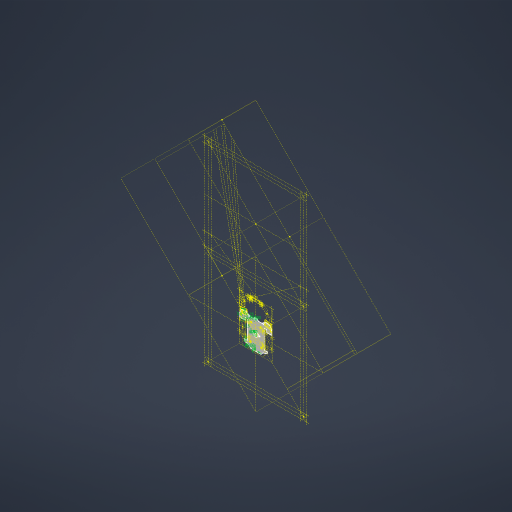
# Autodesk Inventor part: circuit
Saved by Autodesk Inventor 2023.5 (Build 275446000, 446)
## iProperties
Created: 2025-01-11
Part Number: circuit
Material: 一般
Document SubType Name: Modeling
Designer: IshiiLabHonda
Density: 1 g/cm^3
Appearance: 既定
Author: IshiiLabHonda
Autodesk Inventor part; units mm, degrees
ref_plane "YZ Plane" through (0, 0, 0) normal (1, 0, 0) x (0, 1, 0)
ref_plane "XZ Plane" through (0, 0, 0) normal (0, 1, 0) x (-1, 0, 0)
ref_plane "XY Plane" through (0, 0, 0) normal (0, 0, 1) x (1, 0, 0)
derived "chassis.ipt"
sketch "スケッチ1" plane through (0, 0, 0) normal (0, 0, 1) x (1, 0, 0)
  line L0 (0, 0) -> (0, 1) construction
  line L1 (0, 0) -> (1, 0) construction
  line L2 (-90, 90) -> (90, 90) construction
  line L3 (90, 90) -> (90, -90) construction
  line L4 (90, -90) -> (-90, -90) construction
  line L5 (-90, -90) -> (-90, 90) construction
  line L6 (-90, -90) -> (90, 90) construction
  line L7 (-90, 90) -> (90, -90) construction
  line L8 (-84, 96) -> (-84, 84) construction
  line L9 (-84, 84) -> (-96, 84) construction
  line L10 (-96, 84) -> (-96, 96) construction
  line L11 (-96, 96) -> (-84, 84) construction
  line L12 (-84, 96) -> (-96, 84) construction
  line L13 (-96, 96) -> (-84, 96) construction
  line L14 (-96, -96) -> (-96, -84) construction
  line L15 (-84, -96) -> (-96, -96) construction
  line L16 (-96, -96) -> (-84, -84) construction
  line L17 (-96, -84) -> (-84, -96) construction
  line L18 (-84, -84) -> (-84, -96) construction
  line L19 (-96, -84) -> (-84, -84) construction
  line L20 (96, -96) -> (84, -96) construction
  line L21 (96, -84) -> (96, -96) construction
  line L22 (96, -96) -> (84, -84) construction
  line L23 (84, -96) -> (96, -84) construction
  line L24 (84, -84) -> (96, -84) construction
  line L25 (84, -96) -> (84, -84) construction
  line L26 (96, 96) -> (96, 84) construction
  line L27 (84, 96) -> (96, 96) construction
  line L28 (96, 96) -> (84, 84) construction
  line L29 (96, 84) -> (84, 96) construction
  line L30 (84, 84) -> (84, 96) construction
  line L31 (96, 84) -> (84, 84) construction
  line L32 (-84, 84) -> (-84, -84) construction
  line L33 (-96, 84) -> (-96, -84) construction
  line L34 (-84, -84) -> (84, -84) construction
  line L35 (-84, -96) -> (84, -96) construction
  line L36 (96, 84) -> (96, -84) construction
  line L37 (84, 84) -> (84, -84) construction
  line L38 (-84, 96) -> (84, 96) construction
  line L39 (-84, 84) -> (84, 84) construction
  line L40 (-19, 15) -> (19, 15) construction
  line L41 (19, 15) -> (19, -15) construction
  line L42 (19, -15) -> (-19, -15) construction
  line L43 (-19, -15) -> (-19, 15) construction
  line L44 (-19, 15) -> (19, -15) construction
  line L45 (19, 15) -> (-19, -15) construction
  line L46 (-30.25, 11.5) -> (-19, 11.5) construction
  line L47 (-19, -11.5) -> (-30.25, -11.5) construction
  line L48 (-30.25, -11.5) -> (-30.25, 11.5) construction
  line L49 (-30.25, 11.5) -> (-19, -11.5) construction
  line L50 (-19, 11.5) -> (-30.25, -11.5) construction
  line L51 (19, 11.5) -> (30.25, -11.5) construction
  line L52 (19, -11.5) -> (30.25, -11.5) construction
  line L53 (30.25, -11.5) -> (30.25, 11.5) construction
  line L54 (30.25, 11.5) -> (19, 11.5) construction
  line L55 (30.25, 11.5) -> (19, -11.5) construction
  line L56 (-19, -10) -> (19, -10) construction
  line L57 (-19, -12.5) -> (19, -12.5) construction
  line L58 (-19, 12.5) -> (19, 12.5) construction
  line L59 (-19, 10) -> (19, 10) construction
  line L60 (-16.5, -15) -> (-16.5, 15) construction
  line L61 (16.5, -15) -> (16.5, 15) construction
  line L62 (-12.5, -10) -> (-12.5, -15) construction
  line L63 (-16.5, -10) -> (-12.5, -15) construction
  line L64 (-16.5, -15) -> (-12.5, -10) construction
  circle A0 centre (-14.5, -12.5) radius 0.8 construction
  line L65 (12.5, -10) -> (12.5, -15) construction
  line L66 (16.5, -10) -> (12.5, -15) construction
  circle A1 centre (14.5, -12.5) radius 0.8 construction
  line L67 (16.5, -15) -> (12.5, -10) construction
  line L68 (-12.5, 10) -> (-12.5, 15) construction
  line L69 (-16.5, 10) -> (-12.5, 15) construction
  line L70 (-16.5, 15) -> (-12.5, 10) construction
  circle A2 centre (-14.5, 12.5) radius 0.8 construction
  line L71 (12.5, 10) -> (12.5, 15) construction
  line L72 (16.5, 10) -> (12.5, 15) construction
  circle A3 centre (14.5, 12.5) radius 0.8 construction
  line L73 (16.5, 15) -> (12.5, 10) construction
  line L74 (-96, 276) -> (-84, 276) construction
  line L75 (-84, 276) -> (-84, 264) construction
  line L76 (-84, 264) -> (-96, 264) construction
  line L77 (-96, 264) -> (-96, 276) construction
  line L78 (-96, 276) -> (-84, 264) construction
  line L79 (-84, 276) -> (-96, 264) construction
  line L80 (-90, 90) -> (-90, 270) construction
  line L81 (-96, 264) -> (-96, 96) construction
  line L82 (-84, 264) -> (-84, 96) construction
  line L83 (84, 264) -> (84, 96) construction
  line L84 (90, 90) -> (90, 270) construction
  line L85 (96, 264) -> (96, 96) construction
  line L86 (84, 264) -> (96, 264) construction
  line L87 (84, 276) -> (84, 264) construction
  line L88 (96, 276) -> (84, 276) construction
  line L89 (96, 276) -> (84, 264) construction
  line L90 (84, 276) -> (96, 264) construction
  line L91 (96, 264) -> (96, 276) construction
  line L92 (-84, 276) -> (84, 276) construction
  line L93 (-84, 264) -> (84, 264) construction
  line L94 (-90, 270) -> (90, 270) construction
  line L95 (-90, 270) -> (90, 90) construction
  line L96 (-90, 90) -> (90, 270) construction
  circle A4 centre (0, 0) radius 15 construction
  line L97 (-96, 120) -> (96, 120) construction
  line L98 (0, 127.2792) -> (0, -127.2792) construction
  line L99 (-127.2792, 0) -> (127.2792, 0) construction
  line L100 (127.2792, 0) -> (0, -127.2792) construction
  line L101 (0, -127.2792) -> (-127.2792, 0) construction
  line L102 (-127.2792, 0) -> (0, 127.2792) construction
  line L103 (0, 127.2792) -> (127.2792, 0) construction
  line L104 (127.2792, 254.5584) -> (254.5584, 127.2792) construction
  line L105 (254.5584, 127.2792) -> (127.2792, 0) construction
  line L106 (127.2792, 0) -> (0, 127.2792) construction
  line L107 (0, 127.2792) -> (127.2792, 254.5584) construction
  line L108 (-127.2792, 254.5584) -> (0, 127.2792) construction
  line L109 (0, 127.2792) -> (-127.2792, 0) construction
  line L110 (-127.2792, 0) -> (-254.5584, 127.2792) construction
  line L111 (-254.5584, 127.2792) -> (-127.2792, 254.5584) construction
  line L112 (0, 381.8377) -> (127.2792, 254.5584) construction
  line L113 (127.2792, 254.5584) -> (0, 127.2792) construction
  line L114 (0, 127.2792) -> (-127.2792, 254.5584) construction
  line L115 (-127.2792, 254.5584) -> (0, 381.8377) construction
  line L116 (190.9188, 63.6396) -> (63.6396, 190.9188) construction
  line L117 (-190.9188, 190.9188) -> (-63.6396, 63.6396) construction
  line L118 (59.397, -59.397) -> (186.6762, 67.8823) construction
  line L119 (59.397, 186.6762) -> (186.6762, 59.397) construction
  line L120 (63.6396, 190.9188) -> (-63.6396, 318.1981) construction
  line L121 (-186.6762, 186.6762) -> (-59.397, 313.9554) construction
  point P0 (-90, -90)
  point P1 (90, -90)
  point P2 (-24.625, 0)
  point P3 (-84, 120)
  point P4 (84, 120)
  point P5 (0, 0)
sketch "スケッチ5" plane through (0, 0, 0) normal (0, 0, 1) x (1, 0, 0)
  line L0 (0, 0) -> (0, 1) construction
  line L1 (30.25, 11.5) -> (19, 11.5) construction
  line L2 (19, 11.5) -> (30.25, -11.5) construction
  line L3 (30.25, 11.5) -> (19, -11.5) construction
  line L4 (30.25, -11.5) -> (30.25, 11.5) construction
  line L5 (19, -11.5) -> (30.25, -11.5) construction
  line L6 (-90, 90) -> (90, 90) construction
  line L7 (-90, -90) -> (90, 90) construction
  line L8 (-90, 90) -> (90, -90) construction
  line L9 (-84, 84) -> (-84, -84) construction
  line L10 (-96, 84) -> (-96, -84) construction
  line L11 (-90, -90) -> (-90, 90) construction
  line L12 (-84, 84) -> (-96, 84) construction
  line L13 (-96, 84) -> (-96, 96) construction
  line L14 (84, 84) -> (84, -84) construction
  line L15 (90, 90) -> (90, -90) construction
  line L16 (96, 84) -> (84, 84) construction
  line L17 (96, 84) -> (96, -84) construction
  line L18 (90, -90) -> (-90, -90) construction
  line L19 (-84, -84) -> (84, -84) construction
  line L20 (-84, -96) -> (84, -96) construction
  line L21 (-84, -84) -> (-84, -96) construction
  line L22 (-96, -96) -> (-96, -84) construction
  line L23 (-84, -96) -> (-96, -96) construction
  line L24 (-96, -96) -> (-84, -84) construction
  line L25 (-96, -84) -> (-84, -96) construction
  line L26 (-96, -84) -> (-84, -84) construction
  line L27 (0, 0) -> (1, 0) construction
  line L28 (-84, 264) -> (-96, 264) construction
  line L29 (-96, 276) -> (-84, 276) construction
  line L30 (-96, 264) -> (-96, 276) construction
  line L31 (-84, 276) -> (-96, 264) construction
  line L32 (-96, 276) -> (-84, 264) construction
  line L33 (-84, 276) -> (-84, 264) construction
  line L34 (84, -96) -> (84, -84) construction
  line L35 (96, -96) -> (84, -96) construction
  line L36 (96, -84) -> (96, -96) construction
  line L37 (96, -96) -> (84, -84) construction
  line L38 (84, -96) -> (96, -84) construction
  line L39 (84, -84) -> (96, -84) construction
  line L40 (-19, 15) -> (19, 15) construction
  line L41 (19, 15) -> (19, -15) construction
  line L42 (16.5, 15) -> (12.5, 10) construction
  line L43 (12.5, 10) -> (12.5, 15) construction
  line L44 (16.5, 10) -> (12.5, 15) construction
  line L45 (16.5, -15) -> (16.5, 15) construction
  line L46 (-19, 10) -> (19, 10) construction
  line L47 (-19, 12.5) -> (19, 12.5) construction
  circle A0 centre (0, 0) radius 15 construction
  line L48 (-19, -10) -> (19, -10) construction
  line L49 (-19, -12.5) -> (19, -12.5) construction
  line L50 (19, -15) -> (-19, -15) construction
  line L51 (-19, 15) -> (19, -15) construction
  line L52 (19, 15) -> (-19, -15) construction
  line L53 (-16.5, -15) -> (-16.5, 15) construction
  line L54 (-19, -15) -> (-19, 15) construction
  line L55 (-30.25, 11.5) -> (-19, 11.5) construction
  line L56 (-19, -11.5) -> (-30.25, -11.5) construction
  line L57 (-30.25, -11.5) -> (-30.25, 11.5) construction
  line L58 (-30.25, 11.5) -> (-19, -11.5) construction
  line L59 (-19, 11.5) -> (-30.25, -11.5) construction
  line L60 (-12.5, 10) -> (-12.5, 15) construction
  circle A1 centre (-14.5, 12.5) radius 0.8 construction
  line L61 (-16.5, 10) -> (-12.5, 15) construction
  line L62 (-16.5, 15) -> (-12.5, 10) construction
  circle A2 centre (14.5, 12.5) radius 0.8 construction
  line L63 (-84, 96) -> (-96, 84) construction
  line L64 (-96, 96) -> (-84, 96) construction
  line L65 (-84, 96) -> (-84, 84) construction
  line L66 (-96, 96) -> (-84, 84) construction
  line L67 (-96, 264) -> (-96, 96) construction
  line L68 (-84, 264) -> (-84, 96) construction
  line L69 (-84, 96) -> (84, 96) construction
  line L70 (-84, 84) -> (84, 84) construction
  line L71 (84, 84) -> (84, 96) construction
  line L72 (96, 96) -> (96, 84) construction
  line L73 (96, 96) -> (84, 84) construction
  line L74 (96, 84) -> (84, 96) construction
  line L75 (-96, 120) -> (96, 120) construction
  line L76 (84, 96) -> (96, 96) construction
  line L77 (-84, 264) -> (84, 264) construction
  line L78 (84, 264) -> (84, 96) construction
  line L79 (-84, 276) -> (84, 276) construction
  line L80 (96, 264) -> (96, 96) construction
  line L81 (-90, 270) -> (90, 270) construction
  line L82 (-90, 270) -> (90, 90) construction
  line L83 (-90, 90) -> (90, 270) construction
  line L84 (90, 90) -> (90, 270) construction
  line L85 (-90, 90) -> (-90, 270) construction
  line L86 (84, 264) -> (96, 264) construction
  line L87 (96, 276) -> (84, 276) construction
  line L88 (96, 276) -> (84, 264) construction
  line L89 (84, 276) -> (96, 264) construction
  line L90 (96, 264) -> (96, 276) construction
  line L91 (84, 276) -> (84, 264) construction
  circle A3 centre (-14.5, -12.5) radius 0.8 construction
  line L92 (-12.5, -10) -> (-12.5, -15) construction
  line L93 (-16.5, -15) -> (-12.5, -10) construction
  line L94 (12.5, -10) -> (12.5, -15) construction
  circle A4 centre (14.5, -12.5) radius 0.8 construction
  line L95 (16.5, -15) -> (12.5, -10) construction
  line L96 (16.5, -10) -> (12.5, -15) construction
  line L97 (-16.5, -10) -> (-12.5, -15) construction
  line L98 (-12.9773, 53.9269) -> (-10.5199, 55.6476) construction
  line L99 (-8.7991, 53.1902) -> (-12.9773, 53.9269) construction
  circle A5 centre (-10.8882, 53.5585) radius 0.8 construction
  line L100 (-8.7991, 53.1902) -> (-11.2566, 51.4694) construction
  line L101 (-10.5199, 55.6476) -> (-11.2566, 51.4694) construction
  line L102 (-11.2566, 51.4694) -> (-12.9773, 53.9269) construction
  line L103 (-30.25, 44.8844) -> (-31, 44.3592) construction
  line L104 (-12.9471, 57) -> (-30.25, 44.8844) construction
  line L105 (-30.25, 57) -> (-31, 57) construction
  line L106 (-10.5199, 55.6476) -> (-8.7991, 53.1902) construction
  line L107 (-30.25, 57) -> (30.25, 57) construction
  line L108 (-6.2185, 52.5556) -> (-11.543, 48.8274) construction
  line L109 (-11.543, 48.8274) -> (-15.558, 54.5615) construction
  line L110 (-10.2335, 58.2897) -> (-6.2185, 52.5556) construction
  line L111 (1.0005, 57) -> (-30.25, 35.1182) construction
  line L112 (-1.0005, 57) -> (30.25, 35.1182) construction
  line L113 (-19, 15) -> (19, 15) construction
  line L114 (12.5, 10) -> (12.5, 15) construction
  line L115 (-19, 10) -> (19, 10) construction
  circle A6 centre (-14.5, 12.5) radius 0.8 construction
  line L116 (-12.5, 10) -> (-12.5, 15) construction
  line L117 (-16.5, 10) -> (-12.5, 15) construction
  line L118 (-16.5, 15) -> (-12.5, 10) construction
  line L119 (-19, 12.5) -> (19, 12.5) construction
  line L120 (30.25, 57) -> (31, 57) construction
  line L121 (30.25, 11.5) -> (30.25, 57) construction
  line L122 (-6.1403, 52) -> (6.1403, 52) construction
  line L123 (-30.25, 35.1182) -> (-31, 34.593) construction
  line L124 (-30.25, 11.5) -> (-30.25, 57) construction
  line L125 (-6.7921, 53.3748) -> (-12.1165, 49.6465) construction
  line L126 (-10.8882, 53.5585) -> (-10.4294, 52.9032) construction
  line L127 (-10.8882, 53.5585) -> (-10.2329, 54.0174) construction
  line L128 (-6.2185, 52.5556) -> (-15.558, 54.5615) construction
  line L129 (-9.6599, 57.4705) -> (-14.9844, 53.7423) construction
  line L130 (-15.558, 54.5615) -> (-10.2335, 58.2897) construction
  line L131 (-10.2335, 58.2897) -> (-11.543, 48.8274) construction
  line L132 (-30.25, 11.5) -> (-19, 11.5) construction
  line L133 (-30.25, 11.5) -> (-19, -11.5) construction
  line L134 (30.25, 11.5) -> (19, 11.5) construction
  line L135 (30.25, -11.5) -> (30.25, 11.5) construction
  line L136 (19, 11.5) -> (30.25, -11.5) construction
  line L137 (30.25, 11.5) -> (19, -11.5) construction
  line L138 (0, 0) -> (0, 1) construction
  line L139 (0, 0) -> (1, 0) construction
  circle A7 centre (0, 0) radius 7.5 construction
  circle A8 centre (0, 0) radius 15 construction
  line L140 (-16.5, -15) -> (-16.5, 15) construction
  circle A9 centre (14.5, 12.5) radius 0.8 construction
  line L141 (-12.5, -10) -> (-12.5, -15) construction
  line L142 (12.5, -10) -> (12.5, -15) construction
  line L143 (16.5, 10) -> (12.5, 15) construction
  line L144 (-16.5, -15) -> (-12.5, -10) construction
  line L145 (16.5, -10) -> (12.5, -15) construction
  line L146 (16.5, 15) -> (12.5, 10) construction
  line L147 (-19, -12.5) -> (19, -12.5) construction
  line L148 (19, -15) -> (-19, -15) construction
  line L149 (-19, 11.5) -> (-30.25, -11.5) construction
  line L150 (19, -11.5) -> (30.25, -11.5) construction
  line L151 (-19, -11.5) -> (-30.25, -11.5) construction
  line L152 (-30.25, -11.5) -> (-30.25, 11.5) construction
  line L153 (16.5, -15) -> (16.5, 15) construction
  line L154 (19, 15) -> (19, -15) construction
  line L155 (-19, -15) -> (-19, 15) construction
  line L156 (-19, 15) -> (19, -15) construction
  line L157 (19, 15) -> (-19, -15) construction
  line L158 (-31, -8.5) -> (31, -8.5) construction
  line L159 (-31, 8.5) -> (31, 8.5) construction
  line L160 (-31, -31) -> (31, -31) construction
  line L161 (-31, 57) -> (-31, -31) construction
  line L162 (31, 57) -> (31, -31) construction
  line L163 (84, -84) -> (96, -84) construction
  line L164 (84, -96) -> (96, -84) construction
  line L165 (96, -96) -> (84, -84) construction
  line L166 (96, -84) -> (96, -96) construction
  line L167 (96, -96) -> (84, -96) construction
  line L168 (-96, 84) -> (-96, -84) construction
  line L169 (-84, 84) -> (-84, -84) construction
  line L170 (-90, -90) -> (-90, 90) construction
  line L171 (-84, -84) -> (84, -84) construction
  line L172 (-84, -96) -> (84, -96) construction
  line L173 (-90, -90) -> (90, 90) construction
  line L174 (90, -90) -> (-90, -90) construction
  line L175 (-90, 90) -> (90, -90) construction
  line L176 (84, 84) -> (84, -84) construction
  line L177 (90, 90) -> (90, -90) construction
  line L178 (96, 84) -> (96, -84) construction
  line L179 (84, -96) -> (84, -84) construction
  line L180 (-19, -10) -> (19, -10) construction
  circle A10 centre (14.5, -12.5) radius 0.8 construction
  line L181 (16.5, -15) -> (12.5, -10) construction
  line L182 (-16.5, -10) -> (-12.5, -15) construction
  line L183 (-84, -84) -> (-84, -96) construction
  line L184 (-96, -84) -> (-84, -84) construction
  line L185 (-84, -96) -> (-96, -96) construction
  line L186 (-96, -96) -> (-84, -84) construction
  line L187 (-96, -84) -> (-84, -96) construction
  line L188 (-96, -96) -> (-96, -84) construction
  circle A11 centre (-14.5, -12.5) radius 0.8 construction
  line L189 (-96, 96) -> (-84, 96) construction
  line L190 (-84, 96) -> (-84, 84) construction
  line L191 (-84, 96) -> (-96, 84) construction
  line L192 (-96, 96) -> (-84, 84) construction
  line L193 (84, 96) -> (96, 96) construction
  line L194 (96, 84) -> (84, 84) construction
  line L195 (96, 96) -> (96, 84) construction
  line L196 (96, 96) -> (84, 84) construction
  line L197 (96, 84) -> (84, 96) construction
  line L198 (-96, 120) -> (96, 120) construction
  line L199 (-84, 96) -> (84, 96) construction
  line L200 (-90, 90) -> (90, 90) construction
  line L201 (-84, 84) -> (-96, 84) construction
  line L202 (-96, 84) -> (-96, 96) construction
  line L203 (-84, 84) -> (84, 84) construction
  line L204 (84, 120) -> (-30.25, 40.0013) construction
  line L205 (-84, 120) -> (30.25, 40.0013) construction
  line L206 (84, 84) -> (84, 96) construction
  line L207 (-84, 264) -> (-96, 264) construction
  line L208 (-90, 90) -> (-90, 270) construction
  line L209 (-96, 264) -> (-96, 96) construction
  line L210 (-84, 264) -> (-84, 96) construction
  line L211 (96, 264) -> (96, 96) construction
  line L212 (84, 264) -> (84, 96) construction
  line L213 (90, 90) -> (90, 270) construction
  line L214 (-90, 90) -> (90, 270) construction
  line L215 (-90, 270) -> (90, 90) construction
  line L216 (-84, 264) -> (84, 264) construction
  line L217 (-90, 270) -> (90, 270) construction
  line L218 (-96, 264) -> (-96, 276) construction
  line L219 (-96, 276) -> (-84, 276) construction
  line L220 (-96, 276) -> (-84, 264) construction
  line L221 (-84, 276) -> (-96, 264) construction
  line L222 (-84, 276) -> (-84, 264) construction
  line L223 (-84, 276) -> (84, 276) construction
  line L224 (84, 264) -> (96, 264) construction
  line L225 (96, 264) -> (96, 276) construction
  line L226 (96, 276) -> (84, 264) construction
  line L227 (96, 276) -> (84, 276) construction
  line L228 (84, 276) -> (96, 264) construction
  line L229 (84, 276) -> (84, 264) construction
  line L230 (-31, 8.5) -> (-19, 8.5) construction
  line L231 (-31, -8.5) -> (-19, -8.5) construction
  line L232 (-19, 8.5) -> (-19, -8.5) construction
  circle A12 centre (0, 0) radius 7.5 construction
  line L233 (31, -8.5) -> (19, -8.5) construction
  line L234 (19, 8.5) -> (19, -8.5) construction
  line L235 (31, 8.5) -> (19, 8.5) construction
  line L236 (31, 8.5) -> (31, 8.5) projected
  line L237 (-31, -8.5) -> (-12.1203, -31) construction
  line L238 (-12.1203, -31) -> (12.1203, -31) construction
  line L239 (31, -8.5) -> (12.1203, -31) construction
  circle A13 centre (-14.5, 12.5) radius 1.05 construction
  circle A14 centre (14.5, 12.5) radius 1.05 construction
  circle A15 centre (-14.5, -12.5) radius 1.05 construction
  circle A16 centre (14.5, -12.5) radius 1.05 construction
  line L240 (-25.25, 26.5) -> (-25.3613, 27.2922) construction
  line L241 (-25.25, 26.5) -> (-24.4578, 26.6113) construction
  circle A17 centre (-25.25, 26.5) radius 0.8 construction
  line L242 (-23.1223, 29.3236) -> (-22.4264, 24.3723) construction
  line L243 (-27.3777, 23.6764) -> (-28.0736, 28.6277) construction
  line L244 (-23.1223, 29.3236) -> (-27.3777, 23.6764) construction
  line L245 (-28.0736, 28.6277) -> (-23.1223, 29.3236) construction
  line L246 (-22.4264, 24.3723) -> (-27.3777, 23.6764) construction
  line L247 (-28.0736, 28.6277) -> (-22.4264, 24.3723) construction
  line L248 (-28.0736, 28.6277) -> (-27.3777, 23.6764) projected
  line L249 (-23.1223, 29.3236) -> (-18.1709, 30.0195) construction
  line L250 (-18.1709, 30.0195) -> (-17.4751, 25.0681) projected
  line L251 (-17.4751, 25.0681) -> (-22.4264, 24.3723) construction
  line L252 (27.3777, 23.6764) -> (22.4264, 24.3723) construction
  line L253 (17.4751, 25.0681) -> (22.4264, 24.3723) construction
  line L254 (18.1709, 30.0195) -> (17.4751, 25.0681) projected
  line L255 (23.1223, 29.3236) -> (18.1709, 30.0195) construction
  line L256 (23.1223, 29.3236) -> (28.0736, 28.6277) construction
  line L257 (28.0736, 28.6277) -> (27.3777, 23.6764) projected
  line L258 (-28.0736, 28.6277) -> (-18.1709, 30.0195) projected
  line L259 (-17.4751, 25.0681) -> (-18.1709, 30.0195) construction
  line L260 (-17.4751, 25.0681) -> (-27.3777, 23.6764) projected
  line L261 (18.1709, 30.0195) -> (28.0736, 28.6277) projected
  line L262 (27.3777, 23.6764) -> (28.0736, 28.6277) construction
  line L263 (27.3777, 23.6764) -> (17.4751, 25.0681) projected
  line L264 (18.1709, 30.0195) -> (17.4751, 25.0681) construction
  line L265 (-9.6771, 59.2897) -> (9.6771, 59.2897) construction
  line L266 (-9.6771, 59.2897) -> (-9.6771, 59.2897) construction
  line L267 (-3.6771, 59.2897) -> (-0.9296, 58.2897) construction
  line L268 (-0.9296, 58.2897) -> (0.9296, 58.2897) construction
  line L269 (0.9296, 58.2897) -> (3.6771, 59.2897) construction
  line L270 (-4.6137, 54.2897) -> (4.6137, 54.2897) construction
  line L271 (-18.1736, 44.795) -> (-4.6137, 54.2897) construction
  line L272 (-31, 8.5) -> (-22.0451, 50.6295) construction
  line L273 (-22.0451, 50.6295) -> (-9.6771, 59.2897) construction
  line L274 (31, 8.5) -> (22.0451, 50.6295) construction
  line L275 (-18.1736, 44.795) -> (-23.6565, 19) construction
  line L276 (18.1736, 44.795) -> (23.6565, 19) construction
  line L277 (-23.6565, 19) -> (23.6565, 19) construction
  line L278 (-17.6308, -20) -> (17.6308, -20) construction
  line L279 (17.6308, -20) -> (11.5077, -26) construction
  line L280 (11.5077, -26) -> (-11.5077, -26) construction
  line L281 (-11.5077, -26) -> (-17.6308, -20) construction
  line L282 (-31, -8.5) -> (-31, -12.5) construction
  line L283 (-31, -12.5) -> (-12.1203, -31) construction
  line L284 (31, -8.5) -> (31, -12.5) construction
  line L285 (31, -12.5) -> (12.1203, -31) construction
  line L286 (-31, 8.5) -> (-31, 26.5) construction
  line L287 (-31, 26.5) -> (-26.3435, 30.4073) construction
  line L288 (31, 26.5) -> (26.3435, 30.4073) construction
  line L289 (31, 8.5) -> (31, 26.5) construction
  line L290 (-8.1203, -31) -> (-6.6203, -29.5) construction
  line L291 (-6.6203, -29.5) -> (6.6203, -29.5) construction
  line L292 (6.6203, -29.5) -> (8.1203, -31) construction
  line L293 (22.0451, 50.6295) -> (9.6771, 59.2897) construction
  line L294 (18.1736, 44.795) -> (4.6137, 54.2897) construction
  line L295 (-23.6565, 19) -> (-24.8255, 13.5) construction
  line L296 (-24.8255, 13.5) -> (-20.8255, 13.5) construction
  line L297 (-20.8255, 13.5) -> (-15.3255, 19) construction
  line L298 (23.6565, 19) -> (24.8255, 13.5) construction
  line L299 (24.8255, 13.5) -> (20.8255, 13.5) construction
  line L300 (20.8255, 13.5) -> (15.3255, 19) construction
  line L301 (-17.6308, -20) -> (-24.2643, -13.5) construction
  line L302 (-24.2643, -13.5) -> (-21.2643, -13.5) construction
  line L303 (-21.2643, -13.5) -> (-11.6308, -20) construction
  line L304 (21.2643, -13.5) -> (11.6308, -20) construction
  line L305 (17.6308, -20) -> (24.2643, -13.5) construction
  line L306 (24.2643, -13.5) -> (21.2643, -13.5) construction
  line L307 (-10.5173, 23.5) -> (-4.5173, 23.5)
  line L308 (-4.5173, 23.5) -> (-2, 26.5)
  line L309 (-2, 26.5) -> (2, 26.5)
  line L310 (2, 26.5) -> (4.5173, 23.5)
  line L311 (4.5173, 23.5) -> (10.5173, 23.5)
  line L312 (0, 0) -> (1, 0) construction
  line L313 (0, 0) -> (0, 1) construction
  line L314 (-30.5, 13) -> (-20, 13)
  line L315 (-20, 13) -> (-20, 17.5)
  line L316 (-20, 17.5) -> (-16, 17.5)
  line L317 (30.5, 13) -> (20, 13)
  line L318 (20, 13) -> (20, 17.5)
  line L319 (20, 17.5) -> (16, 17.5)
  circle A18 centre (0, 0) radius 1.5
  line L320 (-16, 17.5) -> (-16, -18)
  line L321 (16, 17.5) -> (16, -18)
  line L322 (-30.5, 20.6916) -> (-10.5173, 23.5)
  line L323 (30.5, 20.6916) -> (10.5173, 23.5)
  circle A19 centre (-10.1308, -17) radius 0.625 construction
  circle A20 centre (-10.1308, -17) radius 0.8 projected
  circle A21 centre (-10.1308, -17) radius 1.5 projected
  line L324 (-11.6308, -20) -> (-11.6308, -15) construction
  circle A22 centre (10.1308, -17) radius 0.625 construction
  circle A23 centre (10.1308, -17) radius 0.8 projected
  circle A24 centre (10.1308, -17) radius 1.5 projected
  circle A25 centre (-9, 15.5) radius 0.625 construction
  circle A26 centre (-9, 15.5) radius 0.8 projected
  circle A27 centre (-9, 15.5) radius 1.5 projected
  circle A28 centre (9, 15.5) radius 0.625 construction
  circle A29 centre (9, 15.5) radius 0.8 projected
  circle A30 centre (9, 15.5) radius 1.5 projected
  circle A31 centre (-21.0348, 43.3585) radius 0.8 projected
  circle A32 centre (-21.0348, 43.3585) radius 1.5 construction
  circle A33 centre (21.0348, 43.3585) radius 0.8 projected
  circle A34 centre (21.0348, 43.3585) radius 1.5 construction
  circle A35 centre (21.0348, 43.3585) radius 0.475 construction
  line L325 (-10, -28) -> (10, -28)
  line L326 (-16, -18) -> (-21.9172, -18)
  line L327 (-21.9172, -18) -> (-21.9172, -20)
  line L328 (16, -18) -> (21.9172, -18)
  line L329 (21.9172, -18) -> (21.9172, -20)
  line L330 (-12.8008, -24) -> (-19.7299, -22.1434)
  line L331 (-19.7299, -22.1434) -> (-21.9172, -20)
  line L332 (12.8008, -24) -> (19.7299, -22.1434)
  line L333 (19.7299, -22.1434) -> (21.9172, -20)
  line L334 (-30.5, 13) -> (-30.5, 20.6916)
  line L335 (30.5, 13) -> (30.5, 20.6916)
  line L336 (-12.8008, -24) -> (-10, -28)
  line L337 (10, -28) -> (12.8008, -24)
  line L338 (-1.25, 25) -> (1.25, 25)
  line L339 (2, 24.25) -> (2, 24.25)
  line L340 (1.25, 23.5) -> (-1.25, 23.5)
  line L341 (-2, 24.25) -> (-2, 24.25)
  arc A36 (-1.25, 25) -> (-2, 24.25) centre (-1.25, 24.25) ccw
  arc A37 (-2, 24.25) -> (-1.25, 23.5) centre (-1.25, 24.25) ccw
  arc A38 (1.25, 23.5) -> (2, 24.25) centre (1.25, 24.25) ccw
  arc A39 (2, 24.25) -> (1.25, 25) centre (1.25, 24.25) ccw
  line L342 (-30.5, 20.6916) -> (-27.3668, 27.1909)
  line L343 (-27.3668, 27.1909) -> (-18.4543, 28.4435)
  line L344 (-18.4543, 28.4435) -> (-13.651, 23.0596)
  line L345 (30.5, 20.6916) -> (27.3668, 27.1909)
  line L346 (27.3668, 27.1909) -> (18.4543, 28.4435)
  line L347 (18.4543, 28.4435) -> (13.651, 23.0596)
  line L348 (-29.8721, 30.6471) -> (-16.9987, 32.4563) projected
  line L349 (-16.9987, 32.4563) -> (-15.6765, 23.0488) projected
  line L350 (-15.6765, 23.0488) -> (-28.55, 21.2395) projected
  line L351 (-28.55, 21.2395) -> (-29.8721, 30.6471) projected
  line L352 (-22.0451, 50.6295) -> (-18.1736, 44.795) construction
  line L353 (-21.8107, 27.6837) -> (-26, 24.1685) construction
  line L354 (-26, 24.1685) -> (-26, 13.5) construction
  line L355 (-24.8255, 13.5) -> (-26, 13.5) construction
  line L356 (21.8107, 27.6837) -> (26, 24.1685) construction
  line L357 (26, 24.1685) -> (26, 13.5) construction
  line L358 (24.8255, 13.5) -> (26, 13.5) construction
  circle A40 centre (-28.5, 18.5) radius 0.8 projected
  circle A41 centre (-28.5, 18.5) radius 1.5 projected
  circle A42 centre (-28.5, 18.5) radius 0.475 construction
  line L359 (-18.4543, 28.4435) -> (-10.5173, 23.5)
  line L360 (18.4543, 28.4435) -> (10.5173, 23.5)
  circle A43 centre (28.5, 18.5) radius 0.475 construction
  circle A44 centre (28.5, 18.5) radius 0.8 projected
  circle A45 centre (28.5, 18.5) radius 1.5 projected
  line L361 (-12.9471, 57) -> (12.9471, 57) projected
  circle A46 centre (-6.875, 0) radius 0.9
  circle A47 centre (-6.875, 0) radius 0.8 construction
  circle A48 centre (6.875, 0) radius 0.9
  circle A49 centre (6.875, 0) radius 0.8 construction
  circle A50 centre (0, 0) radius 5.75 construction
  circle A51 centre (-6.875, 0) radius 0.625 construction
  circle A52 centre (0, 0) radius 4.25
  line L362 (29.8721, 30.6471) -> (16.9987, 32.4563) projected
  line L363 (16.9987, 32.4563) -> (15.6765, 23.0488) projected
  line L364 (15.6765, 23.0488) -> (28.55, 21.2395) projected
  line L365 (28.55, 21.2395) -> (29.8721, 30.6471) projected
  line L366 (-23.4801, 43.8782) -> (-18.5894, 42.8387) construction
  line L367 (-20.1093, 47.7123) -> (-28.4441, 8.5) construction
  line L368 (-13.2559, 53.976) -> (-10.4708, 55.9262) projected
  line L369 (-10.4708, 55.9262) -> (-8.5206, 53.1411) projected
  line L370 (-8.5206, 53.1411) -> (-11.3057, 51.1909) projected
  line L371 (-11.3057, 51.1909) -> (-13.2559, 53.976) projected
  line L372 (-13.2559, 53.976) -> (-8.5206, 53.1411) construction
  line L373 (-10.4708, 55.9262) -> (-11.3057, 51.1909) construction
  line L374 (13.2559, 53.976) -> (10.4708, 55.9262) projected
  line L375 (11.3057, 51.1909) -> (13.2559, 53.976) projected
  line L376 (8.5206, 53.1411) -> (11.3057, 51.1909) projected
  line L377 (10.4708, 55.9262) -> (8.5206, 53.1411) projected
  circle A53 centre (-10.8882, 53.5585) radius 1.05 projected
  circle A54 centre (10.8882, 53.5585) radius 1.05 projected
  point P0 (-90, -90)
  point P1 (90, -90)
  point P2 (-24.625, 0)
  point P3 (-8.226, 55.4227)
  point P4 (-5.9733, 57)
  point P5 (0, 61.1826)
  point P6 (-24.625, 0)
  point P7 (-90, -90)
  point P8 (90, -90)
  point P9 (-5.9733, 57)
  point P10 (5.9733, 57)
  point P11 (12.9773, 53.9269)
  point P12 (8.7991, 53.1902)
  point P13 (28.2604, 20.217)
  point P14 (29.75, 18.3552)
  point P15 (-2, 25)
  point P16 (-2, 23.5)
  point P17 (-2, 24.25)
  point P18 (2, 24.25)
  point P19 (13.651, 23.0596)
  point P20 (20.4797, 27.6588)
  point P21 (29.7346, 22.6965)
  point P22 (-20.4797, 27.6588)
  point P23 (-29.7346, 22.6965)
  point P24 (17.855, 27.7717)
  point P25 (-17.855, 27.7717)
  point P26 (-27.7577, 26.38)
  point P27 (-17.901, 28.0988)
  point P28 (-28.9305, 23.9472)
  point P29 (-16.057, 25.7564)
  point P30 (16.2409, 27.0649)
  point P31 (28.9305, 23.9472)
  point P32 (27.7577, 26.38)
  point P33 (17.901, 28.0988)
  point P34 (-16.2409, 27.0649)
  dimension "d4" = 3
  dimension "d22" = 0.5
  dimension "d23" = 2.5
  dimension "d24" = 3
  dimension "d25" = 1
  dimension "d26" = 2
  dimension "d27" = 3
  dimension "d28" = 125
  dimension "d29" = 140
  dimension "d30" = 20
  dimension "d31" = 4
  dimension "d32" = 4
  dimension "d33" = 1.5
  dimension "d34" = 1.5
  dimension "d35" = 0.75
  dimension "d36" = 6
  dimension "d37" = 130
  dimension "d38" = 4
  dimension "d43" = 6
  dimension "d46" = 4
  dimension "d52" = 9
  dimension "d57" = 1.5
  dimension "d58" = 0.5
  dimension "d61" = 6
  dimension "d75" = 1.6
  dimension "d76" = 0.1
  dimension "d78" = 1.25
  dimension "d79" = 0.5
  dimension "d82" = 1.5
  dimension "d83" = 8.5
  constraints: 80 end point, 20 horizontal alignment, 12 centre point, 12 parallel, 8 point on circle, 8 tangent, 6 coincident, 6 point on line, 5 equal radius, 3 horizontal, 2 symmetric about line, 2 vertical, 1 collinear, 1 perpendicular, 38 other
  measures "d4" diameter of A18
  measures "d22" distance between parallel lines of L53 L320
  measures "d25" distance between parallel lines of L283 L331
  measures "d26" distance of L326.end L327.end
  measures "d27" distance between parallel lines of L238 L325
  measures "d28" angle of L336 L325
  measures "d29" angle of L336 L330
  measures "d30" distance of L325.start L325.end
  measures "d31" distance from line of L330.start L325
  measures "d32" distance of L308.end L309.end
  measures "d33" distance between parallel lines of L338 L309
  measures "d34" distance of point (-2, 23.5) point (-2, 25)
  measures "d35" radius of A36
  measures "d36" distance between parallel lines of L316 L307
  measures "d37" angle of L309 L308
  measures "d38" distance of L339.start L341.end
  measures "d43" distance of L307.start L307.end
  measures "d46" distance of L315.end L316.end
  measures "d52" distance of L342.end L343.end
  measures "d57" distance between parallel lines of L55 L314
  measures "d58" distance between parallel lines of L286 L334
  measures "d61" distance between parallel lines of L322 L343
  measures "d75" diameter of A47
  measures "d76" radial gap between concentric circles of A47 A46
  measures "d78" diameter of A51
  measures "d82" radial gap between concentric circles of A50 A52
  measures "d83" diameter of A52
extrude "押し出し1" add sketch "スケッチ5" against normal blind 0.8 contours L322 L307 L308 L309 L310 L311 L323 L335 L317 L318 L319 L321 L328 L329 L333 L332 L337 L325 L336 L330 L331 L327 L326 L320 L316 L315 L314 L334 | A18 | A20 | A21 | A23 | A24 | A26 | A27 | A29 | A30 | L338 A39 A38 L340 A37 A36 | A40 | A41 | A44 | A45 | A46 | A48 | A52
extrude "押し出し5" cut sketch "スケッチ5" against normal blind 0.8 contours A20 | A23 | A26 | A29
extrude "押し出し8" add sketch "スケッチ5" against normal blind 0.8 contours L322 L307 L308 L309 L310 L311 L323 L335 L317 L318 L319 L321 L328 L329 L333 L332 L337 L325 L336 L330 L331 L327 L326 L320 L316 L315 L314 L334 | A18 | A20 | A21 | A23 | A24 | A26 | A27 | A29 | A30 | L338 A39 A38 L340 A37 A36 | A40 | A41 | A44 | A45 | A46 | A48 | A52
extrude "押し出し10" cut sketch "スケッチ5" against normal blind 0.8 contours A20 | A23 | A26 | A29 | L338 A39 A38 L340 A37 A36
extrude "押し出し12" add sketch "スケッチ5" against normal blind 0.8 contours L342 L343 L344 L250 L260 L248 | L248 L260 L250 L344 L349 L350 L351 L342 | L351 L350 L349 L344 L322 L342 | L347 L363 L364 L365 L345 L323 | L347 L254 L263 L257 L345 L365 L364 L363 | L347 L346 L345 L257 L263 L254
extrude "押し出し14" cut sketch "スケッチ5" against normal blind 1 contours A40
extrude "押し出し15" add sketch "スケッチ5" against normal blind 0.8 contours L359 L349 L344 L250 | L250 L344 L359 | L359 L322 L344 L349 | L360 L363 L347 L323 | L360 L254 L347 L363 | L360 L347 L254
extrude "押し出し16" cut sketch "スケッチ5" against normal blind 0.8 contours A44
extrude "押し出し17" cut sketch "スケッチ5" against normal blind 0.1 contours L342 L343 L344 L250 L260 L248 | L250 L344 L359
chamfer "面取り1" distance 0.8 angle 45 4 edges at (-20, 17.5, -0.4) (-16, 17.5, -0.4) (16, 17.5, -0.4) (20, 17.5, -0.4)
chamfer "面取り2" distance 0.8 angle 45 4 edges at (-20, 13, -0.4) (-30.5, 13, -0.4) (20, 13, -0.4) (30.5, 13, -0.4)
mirror "ミラー1" about plane through (0, 0, 0) normal (1, 0, 0) of "押し出し17"
extrude "押し出し18" cut sketch "スケッチ5" against normal blind 5 contours A18 | A46 | A48
extrude "押し出し19" cut sketch "スケッチ5" against normal blind 0.2 contours L248 L260 L250 L344 L349 L350 L351 L342 | L359 L349 L344 L250 | L360 L254 L347 L363 | L347 L254 L263 L257 L345 L365 L364 L363
chamfer "面取り3" distance 1 angle 45 2 edges at (-16, -18, -0.4) (16, -18, -0.4)
sketch "スケッチ4" plane through (0, 0, 0) normal (0, 0, 1) x (1, 0, 0)
  line L0 (-84, 264) -> (-96, 264) construction
  line L1 (-90, 90) -> (-90, 270) construction
  line L2 (-96, 264) -> (-96, 96) construction
  line L3 (-96, 96) -> (-84, 96) construction
  line L4 (-84, 96) -> (-84, 84) construction
  line L5 (-84, 96) -> (-96, 84) construction
  line L6 (-96, 96) -> (-84, 84) construction
  line L7 (-84, 264) -> (-84, 96) construction
  line L8 (-84, 84) -> (-96, 84) construction
  line L9 (84, -84) -> (96, -84) construction
  line L10 (84, -96) -> (96, -84) construction
  line L11 (96, -96) -> (84, -84) construction
  line L12 (96, -84) -> (96, -96) construction
  line L13 (96, -96) -> (84, -96) construction
  line L14 (0, 0) -> (0, 1) construction
  line L15 (0, 0) -> (1, 0) construction
  line L16 (16.5, 15) -> (12.5, 10) construction
  line L17 (-96, 84) -> (-96, -84) construction
  line L18 (-84, 84) -> (-84, -84) construction
  line L19 (-90, -90) -> (-90, 90) construction
  line L20 (-90, 90) -> (90, 90) construction
  line L21 (-84, -84) -> (84, -84) construction
  line L22 (-84, -96) -> (84, -96) construction
  line L23 (-90, -90) -> (90, 90) construction
  line L24 (90, -90) -> (-90, -90) construction
  line L25 (-90, 90) -> (90, -90) construction
  line L26 (84, 84) -> (84, -84) construction
  line L27 (90, 90) -> (90, -90) construction
  line L28 (96, 84) -> (96, -84) construction
  line L29 (-96, 84) -> (-96, 96) construction
  line L30 (-84, -84) -> (-84, -96) construction
  line L31 (-96, -84) -> (-84, -84) construction
  line L32 (-84, -96) -> (-96, -96) construction
  line L33 (-96, -96) -> (-84, -84) construction
  line L34 (-96, -84) -> (-84, -96) construction
  line L35 (-96, -96) -> (-96, -84) construction
  line L36 (84, -96) -> (84, -84) construction
  line L37 (-19, -15) -> (-19, 15) construction
  line L38 (-30.25, 11.5) -> (-19, 11.5) construction
  line L39 (-19, -11.5) -> (-30.25, -11.5) construction
  line L40 (-19, 11.5) -> (-30.25, -11.5) construction
  line L41 (-30.25, 11.5) -> (-19, -11.5) construction
  line L42 (-30.25, -11.5) -> (-30.25, 11.5) construction
  line L43 (12.5, 10) -> (12.5, 15) construction
  circle A0 centre (14.5, 12.5) radius 0.8 construction
  line L44 (30.25, 11.5) -> (19, 11.5) construction
  line L45 (16.5, 10) -> (12.5, 15) construction
  circle A1 centre (14.5, -12.5) radius 0.8 construction
  line L46 (16.5, -15) -> (12.5, -10) construction
  line L47 (16.5, -10) -> (12.5, -15) construction
  line L48 (12.5, -10) -> (12.5, -15) construction
  circle A2 centre (-14.5, -12.5) radius 0.8 construction
  line L49 (-12.5, -10) -> (-12.5, -15) construction
  line L50 (-16.5, -15) -> (-12.5, -10) construction
  line L51 (-16.5, -10) -> (-12.5, -15) construction
  line L52 (96, 84) -> (84, 84) construction
  line L53 (96, 96) -> (96, 84) construction
  line L54 (84, 96) -> (96, 96) construction
  line L55 (96, 96) -> (84, 84) construction
  line L56 (84, 84) -> (84, 96) construction
  line L57 (96, 84) -> (84, 96) construction
  line L58 (-96, 264) -> (-96, 276) construction
  line L59 (-84, 276) -> (-84, 264) construction
  line L60 (-96, 276) -> (-84, 276) construction
  line L61 (-96, 276) -> (-84, 264) construction
  line L62 (-84, 276) -> (-96, 264) construction
  line L63 (-84, 84) -> (84, 84) construction
  line L64 (-84, 96) -> (84, 96) construction
  line L65 (84, 264) -> (84, 96) construction
  line L66 (90, 90) -> (90, 270) construction
  line L67 (-90, 90) -> (90, 270) construction
  line L68 (-90, 270) -> (90, 90) construction
  line L69 (96, 264) -> (96, 96) construction
  line L70 (-96, 120) -> (96, 120) construction
  line L71 (-84, 264) -> (84, 264) construction
  line L72 (-84, 276) -> (84, 276) construction
  line L73 (-90, 270) -> (90, 270) construction
  line L74 (84, 276) -> (84, 264) construction
  line L75 (84, 264) -> (96, 264) construction
  line L76 (96, 264) -> (96, 276) construction
  line L77 (96, 276) -> (84, 264) construction
  line L78 (96, 276) -> (84, 276) construction
  line L79 (84, 276) -> (96, 264) construction
  line L80 (-19, 15) -> (19, 15) construction
  line L81 (19, 15) -> (19, -15) construction
  line L82 (19, -15) -> (-19, -15) construction
  circle A3 centre (-14.5, 12.5) radius 0.8 construction
  line L83 (-16.5, 10) -> (-12.5, 15) construction
  line L84 (-12.5, 10) -> (-12.5, 15) construction
  line L85 (-16.5, 15) -> (-12.5, 10) construction
  circle A4 centre (0, 0) radius 15 construction
  line L86 (-19, 10) -> (19, 10) construction
  line L87 (-19, 12.5) -> (19, 12.5) construction
  line L88 (-19, 15) -> (19, -15) construction
  line L89 (19, 15) -> (-19, -15) construction
  line L90 (-19, -10) -> (19, -10) construction
  line L91 (-19, -12.5) -> (19, -12.5) construction
  line L92 (16.5, -15) -> (16.5, 15) construction
  line L93 (19, 11.5) -> (30.25, -11.5) construction
  line L94 (19, -11.5) -> (30.25, -11.5) construction
  line L95 (30.25, -11.5) -> (30.25, 11.5) construction
  line L96 (30.25, 11.5) -> (19, -11.5) construction
  line L97 (-16.5, -15) -> (-16.5, 15) construction
  line L98 (-84, 120) -> (30.25, 40.0013) construction
  line L99 (84, 120) -> (-30.25, 40.0013) construction
  line L100 (-30.25, 57) -> (30.25, 57) construction
  line L101 (1.0005, 57) -> (-30.25, 35.1182) construction
  line L102 (-1.0005, 57) -> (30.25, 35.1182) construction
  line L103 (-12.9471, 57) -> (-30.25, 44.8844) construction
  line L104 (-10.2335, 58.2897) -> (-6.2185, 52.5556) construction
  line L105 (-6.2185, 52.5556) -> (-11.543, 48.8274) construction
  line L106 (-11.543, 48.8274) -> (-15.558, 54.5615) construction
  line L107 (-15.558, 54.5615) -> (-10.2335, 58.2897) construction
  line L108 (-10.2335, 58.2897) -> (-11.543, 48.8274) construction
  line L109 (-6.2185, 52.5556) -> (-15.558, 54.5615) construction
  line L110 (-9.6599, 57.4705) -> (-14.9844, 53.7423) construction
  line L111 (-6.7921, 53.3748) -> (-12.1165, 49.6465) construction
  line L112 (-10.8882, 53.5585) -> (-10.2329, 54.0174) construction
  line L113 (-10.8882, 53.5585) -> (-10.4294, 52.9032) construction
  line L114 (-10.5199, 55.6476) -> (-8.7991, 53.1902) construction
  line L115 (-8.7991, 53.1902) -> (-11.2566, 51.4694) construction
  line L116 (-11.2566, 51.4694) -> (-12.9773, 53.9269) construction
  line L117 (-12.9773, 53.9269) -> (-10.5199, 55.6476) construction
  line L118 (-10.5199, 55.6476) -> (-11.2566, 51.4694) construction
  line L119 (-8.7991, 53.1902) -> (-12.9773, 53.9269) construction
  circle A5 centre (-10.8882, 53.5585) radius 0.8 construction
  line L120 (-30.25, 11.5) -> (-30.25, 57) construction
  line L121 (30.25, 11.5) -> (30.25, 57) construction
  line L122 (-6.1403, 52) -> (6.1403, 52) construction
  line L123 (-31, 57) -> (-31, -31) construction
  line L124 (31, 57) -> (31, -31) construction
  line L125 (-30.25, 57) -> (-31, 57) construction
  line L126 (30.25, 57) -> (31, 57) construction
  line L127 (-31, 8.5) -> (31, 8.5) construction
  line L128 (-31, -8.5) -> (31, -8.5) construction
  circle A6 centre (0, 0) radius 7.5 construction
  line L129 (-31, -31) -> (31, -31) construction
  line L130 (-30.25, 44.8844) -> (-31, 44.3592) construction
  line L131 (-30.25, 35.1182) -> (-31, 34.593) construction
  line L132 (-25.25, 26.5) -> (-25.3613, 27.2922) construction
  line L133 (-25.25, 26.5) -> (-24.4578, 26.6113) construction
  line L134 (-28.0736, 28.6277) -> (-23.1223, 29.3236) construction
  line L135 (-23.1223, 29.3236) -> (-22.4264, 24.3723) construction
  line L136 (-22.4264, 24.3723) -> (-27.3777, 23.6764) construction
  line L137 (-27.3777, 23.6764) -> (-28.0736, 28.6277) construction
  line L138 (-28.0736, 28.6277) -> (-22.4264, 24.3723) construction
  line L139 (-23.1223, 29.3236) -> (-27.3777, 23.6764) construction
  circle A7 centre (-25.25, 26.5) radius 0.8 construction
  line L140 (-25.25, 57) -> (-25.25, -31) construction
  line L141 (-96, 180) -> (96, 180) construction
  line L142 (-25.3613, 27.2922) -> (-64.8788, 308.4736) construction
  line L143 (-186.6762, 186.6762) -> (-59.397, 313.9554) construction
  line L144 (59.397, 186.6762) -> (186.6762, 59.397) construction
  line L145 (-25.25, 26.5) -> (-79.6192, 293.7332) construction
  line L146 (-25.25, 26.5) -> (-46.8888, 301.4473) construction
  line L147 (63.6396, 190.9188) -> (-63.6396, 318.1981) construction
  line L148 (10.8882, 53.5585) -> (10.2329, 54.0174) construction
  line L149 (10.8882, 53.5585) -> (10.4294, 52.9032) construction
  circle A8 centre (10.8882, 53.5585) radius 0.8 construction
  line L150 (12.9773, 53.9269) -> (10.5199, 55.6476) construction
  line L151 (10.5199, 55.6476) -> (11.2566, 51.4694) construction
  line L152 (11.2566, 51.4694) -> (12.9773, 53.9269) construction
  line L153 (11.543, 48.8274) -> (15.558, 54.5615) construction
  line L154 (8.7991, 53.1902) -> (11.2566, 51.4694) construction
  line L155 (6.7921, 53.3748) -> (12.1165, 49.6465) construction
  line L156 (10.5199, 55.6476) -> (8.7991, 53.1902) construction
  line L157 (6.2185, 52.5556) -> (15.558, 54.5615) construction
  line L158 (9.6599, 57.4705) -> (14.9844, 53.7423) construction
  line L159 (8.7991, 53.1902) -> (12.9773, 53.9269) construction
  line L160 (6.2185, 52.5556) -> (11.543, 48.8274) construction
  line L161 (10.2335, 58.2897) -> (6.2185, 52.5556) construction
  line L162 (15.558, 54.5615) -> (10.2335, 58.2897) construction
  line L163 (10.2335, 58.2897) -> (11.543, 48.8274) construction
  line L164 (-23.1223, 29.3236) -> (-18.1709, 30.0195) construction
  line L165 (-18.1709, 30.0195) -> (-17.4751, 25.0681) construction
  line L166 (-17.4751, 25.0681) -> (-22.4264, 24.3723) construction
  line L167 (-23.1223, 29.3236) -> (-28.0736, 28.6277) construction
  line L168 (-28.0736, 28.6277) -> (-27.3777, 23.6764) construction
  line L169 (-27.3777, 23.6764) -> (-22.4264, 24.3723) construction
  line L170 (23.1223, 29.3236) -> (28.0736, 28.6277) construction
  line L171 (27.3777, 23.6764) -> (22.4264, 24.3723) construction
  line L172 (17.4751, 25.0681) -> (22.4264, 24.3723) construction
  line L173 (27.3777, 23.6764) -> (28.0736, 28.6277) construction
  line L174 (18.1709, 30.0195) -> (17.4751, 25.0681) construction
  line L175 (23.1223, 29.3236) -> (18.1709, 30.0195) construction
  line L176 (28.0736, 28.6277) -> (27.3777, 23.6764) construction
  line L177 (23.1223, 29.3236) -> (27.3777, 23.6764) construction
  line L178 (22.4264, 24.3723) -> (28.0736, 28.6277) construction
  line L179 (-20.2987, 27.1959) -> (-60.4518, 312.9005) construction
  line L180 (-20.2987, 27.1959) -> (-41.4551, 296.0135) construction
  line L181 (-20.2987, 27.1959) -> (-75.3873, 297.9651) construction
  line L182 (-23.1223, 29.3236) -> (-17.4751, 25.0681) construction
  line L183 (-22.4264, 24.3723) -> (-18.1709, 30.0195) construction
  line L184 (-15.558, 54.5615) -> (-18.0155, 52.8407) construction
  line L185 (-18.0155, 52.8407) -> (-14.0004, 47.1067) construction
  line L186 (-14.0004, 47.1067) -> (-11.543, 48.8274) construction
  point P0 (90, -90)
  point P1 (-90, -90)
  point P2 (-24.625, 0)
  point P3 (0, 61.1826)
  point P4 (-5.9733, 57)
  point P5 (-8.226, 55.4227)
  point P6 (0, 180)
  point P7 (8.226, 55.4227)
  constraints: 2 other
